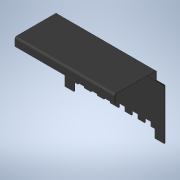
# Autodesk Inventor part: controlbox_cover
Saved by Autodesk Inventor 2020 (Build 240168000, 168)
## iProperties
Created: 2020-06-02
Part Number: controlbox_cover
Material: Generic
Document SubType Name: Modeling
Designer: Gebruiker
Density: 1 g/cm^3
Appearance: Default
Author: Gebruiker
Autodesk Inventor part; units mm, degrees
ref_plane "YZ Plane" through (0, 0, 0) normal (1, 0, 0) x (0, 1, 0)
ref_plane "XZ Plane" through (0, 0, 0) normal (0, 1, 0) x (-1, 0, 0)
ref_plane "XY Plane" through (0, 0, 0) normal (0, 0, 1) x (1, 0, 0)
sketch "Sketch1" plane through (0, 0, 0) normal (1, 0, 0) x (0, 1, 0)
  line L0 (60.5, 1.15) -> (-60.5, 1.15)
  line L1 (-60.5, 1.15) -> (-60.5, -1.15)
  line L2 (-60.5, -1.15) -> (60.5, -1.15)
  line L3 (60.5, -1.15) -> (60.5, 1.15)
  line L4 (60.5, 1.15) -> (-60.5, -1.15) construction
  line L5 (-60.5, 1.15) -> (60.5, -1.15) construction
  line L6 (60.5, -1.15) -> (81.7132, 20.0632)
  line L7 (60.5, -1.15) -> (90.5, -1.15) construction
  line L8 (81.7132, 20.0632) -> (80.0869, 21.6895)
  line L9 (80.0869, 21.6895) -> (59.5288, 1.1315)
  line L10 (80.0869, 21.6895) -> (100.0869, 21.6895)
  line L11 (100.0869, 21.6895) -> (100.0869, 19.3895)
  line L12 (100.0869, 19.3895) -> (81.0395, 19.3895)
  line L13 (100.0869, 19.3895) -> (102.3869, 19.3895)
  line L14 (102.3869, 19.3895) -> (102.3869, 120.8895)
  line L15 (102.3869, 120.8895) -> (100.0869, 120.8895)
  line L16 (100.0869, 120.8895) -> (100.0869, 19.3895)
  line L17 (102.3869, 120.8895) -> (82.3869, 120.8895)
  line L18 (82.3869, 120.8895) -> (82.3869, 116.8895)
  line L19 (82.3869, 116.8895) -> (102.3869, 116.8895)
  line L20 (102.3869, 116.8895) -> (102.3869, 120.8895)
  point P0 (0, 0)
  point P1 (59.5473, 1.15)
  point P2 (100.0869, 116.8895)
  point P3 (100.0869, 21.6895)
  dimension "d0" = 121
  dimension "d1" = 2.3
  dimension "d2" = 30
  dimension "d3" = 45
  dimension "d4" = 2.3
  dimension "d5" = 20
  dimension "d6" = 2.3
  dimension "d7" = 2.3
  dimension "d8" = 101.5
  dimension "d9" = 20
  dimension "d10" = 4
  constraints: 42 end point, 7 perpendicular, 6 parallel, 5 horizontal, 2 midpoint, 2 point on line, 1 equal length
  measures "d0" distance of L2.end L1.end
  measures "d1" distance of L1.end L0.end
  measures "d2" distance of L2.end L6.end
  measures "d3" angle of L7 L6
  measures "d4" distance of L6.end L8.end
  measures "d5" distance of L8.end L10.end
  measures "d6" distance of L10.end L11.end
  measures "d7" distance of L15.end L14.end
  measures "d8" distance of L14.end L13.end
  measures "d9" distance of L19.end L18.end
  measures "d10" distance of L18.end L17.end
extrude "Extrusion1" add sketch "Sketch1" against normal blind 239
fillet "Fillet1" radius 4 1 edges at (-119.5, 60.5, -1.15)
fillet "Fillet2" radius 4 5 edges at (-119.5, 59.5473, 1.15) (-119.5, 81.0395, 19.3895) (-119.5, 80.0869, 21.6895) (-119.5, 102.3869, 120.8895) (-119.5, 100.0869, 116.8895)
sketch "Sketch2" plane through (0, -60.5, -1.15) normal (0, 0, -1) x (-1, 0, 0)
  line L0 (22, -20) -> (217, -20)
  line L1 (217, -20) -> (217, 20)
  line L2 (217, 20) -> (22, 20)
  line L3 (22, 20) -> (22, -20)
  line L4 (0, 0) -> (239, 0) projected
  line L5 (22, -20) -> (217, 20) construction
  line L6 (217, -20) -> (22, 20) construction
  line L7 (239, 119.3431) -> (239, 0) projected
  line L8 (0, 0) -> (0, 119.3431) projected
  line L9 (119.5, 20) -> (119.5, 119.3431) construction
  line L10 (119.5, 119.3431) -> (119.5, 0) construction
  line L11 (32, 20) -> (47, 20) construction
  line L12 (47, 20) -> (47, 30)
  line L13 (47, 30) -> (32, 30)
  line L14 (32, 30) -> (32, 20)
  line L15 (32, 20) -> (47, 20) construction
  line L16 (55.3012, 20) -> (70.3012, 20)
  line L17 (94.5, 20) -> (109.5, 20)
  line L18 (109.5, 20) -> (109.5, 30)
  line L19 (109.5, 30) -> (94.5, 30)
  line L20 (94.5, 30) -> (94.5, 20)
  line L21 (63.25, 20) -> (78.25, 20)
  line L22 (78.25, 20) -> (78.25, 30)
  line L23 (78.25, 30) -> (63.25, 30)
  line L24 (63.25, 30) -> (63.25, 20)
  line L25 (47, 30) -> (63.25, 30) construction
  line L26 (78.25, 30) -> (94.5, 30) construction
  line L27 (192, 20) -> (192, 30)
  line L28 (192, 30) -> (207, 30)
  line L29 (207, 30) -> (207, 20)
  line L30 (129.5, 20) -> (129.5, 30)
  line L31 (129.5, 30) -> (144.5, 30)
  line L32 (144.5, 30) -> (144.5, 20)
  line L33 (160.75, 20) -> (160.75, 30)
  line L34 (160.75, 30) -> (175.75, 30)
  line L35 (175.75, 30) -> (175.75, 20)
  point P0 (0, 60.5)
  point P1 (22, 0)
  point P2 (217, 0)
  point P3 (109.5, 20)
  point P4 (192, 20)
  point P5 (207, 20)
  point P6 (160.75, 20)
  dimension "d15" = 195
  dimension "d16" = 40
  dimension "d19" = 22
  dimension "d20" = 22
  dimension "d21" = 15
  dimension "d22" = 10
  dimension "d25" = 15
  dimension "d26" = 10
  dimension "d27" = 10
  dimension "d28" = 10
  dimension "d31" = 15
  dimension "d32" = 10
  constraints: 66 end point, 12 symmetric about line, 8 parallel, 5 horizontal, 5 perpendicular, 4 midpoint, 4 point on line, 2 collinear, 1 vertical
  measures "d15" distance of L2.end L1.end
  measures "d16" distance of L1.end L0.end
  measures "d19" distance from line of L7 L1.end
  measures "d20" distance from line of L8 L2.end
  measures "d21" distance of L13.end L12.end
  measures "d22" distance of L12.end L11.end
  measures "d25" distance of L19.end L18.end
  measures "d26" distance of L18.end L17.end
  measures "d27" distance of L11.start L2.end
  measures "d28" distance of L9.start L17.end
  measures "d31" distance of L23.end L22.end
  measures "d32" distance of L22.end L21.end
extrude "Extrusion2" cut sketch "Sketch2" against normal blind 10 contours L3 L2 L1 L4 | L14 L13 L12 L2 | L2 L27 L28 L29 | L2 L33 L34 L35 | L24 L23 L22 L2 | L2 L30 L31 L32 | L20 L19 L18 L2
body "Solid1"
